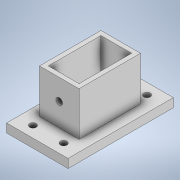
# Autodesk Inventor part: Lens Holder
Saved by Autodesk Inventor 2022 (Build 260153000, 153)
## iProperties
Created: 2023-09-18
Part Number: Lens Holder
Material: Generic
Document SubType Name: Modeling
Designer: fouad
Density: 1 g/cm^3
Appearance: Default
Author: fouad
Autodesk Inventor part; units mm, degrees
ref_plane "YZ Plane" through (0, 0, 0) normal (1, 0, 0) x (0, 1, 0)
ref_plane "XZ Plane" through (0, 0, 0) normal (0, 1, 0) x (-1, 0, 0)
ref_plane "XY Plane" through (0, 0, 0) normal (0, 0, 1) x (1, 0, 0)
sketch "Sketch1" plane through (0, 0, 0) normal (0, 1, 0) x (-1, 0, 0)
  line L0 (7.074, 9.2769) -> (0.074, 9.2769)
  line L1 (0.074, 9.2769) -> (0.074, -2.7231)
  line L2 (0.074, -2.7231) -> (7.074, -2.7231)
  line L3 (7.074, -2.7231) -> (7.074, 9.2769)
  line L4 (5.324, 6.2769) -> (1.824, 6.2769)
  line L5 (1.824, 6.2769) -> (1.824, 0.2769)
  line L6 (1.824, 0.2769) -> (5.324, 0.2769)
  line L7 (5.324, 0.2769) -> (5.324, 6.2769)
  point P0 (0, 0)
  dimension "d0" = 7
  dimension "d1" = 12
  dimension "d28" = 1.75
  dimension "d29" = 1.75
  dimension "d30" = 3
  dimension "d31" = 3
  constraints: 16 end point, 4 parallel, 2 horizontal, 2 perpendicular
  measures "d0" distance of L2.end L1.end
  measures "d1" distance of L1.end L0.end
  measures "d28" distance between parallel lines of L7 L3
  measures "d29" distance between parallel lines of L1 L5
  measures "d30" distance between parallel lines of L6 L2
  measures "d31" distance between parallel lines of L0 L4
extrude "Extrusion1" add sketch "Sketch1" along normal blind 1
sketch "Sketch3" plane through (0, 1, 0) normal (0, 1, 0) x (1, 0, 0)
  circle A0 centre (-5.324, -8.0269) radius 0.375
  line L0 (-7.074, -9.2769) -> (-0.074, -9.2769) projected
  line L1 (-7.074, 2.7231) -> (-7.074, -9.2769) projected
  circle A1 centre (-1.824, -8.0269) radius 0.375
  circle A2 centre (-5.324, 1.4731) radius 0.375
  circle A3 centre (-1.824, 1.4731) radius 0.375
  point P0 (0, 0)
  dimension "d8" = 0.75
  dimension "d9" = 1.25
  dimension "d10" = 1.75
  dimension "d13" = 3.5
  dimension "d16" = 9.5
  constraints: 4 centre point, 1 horizontal, 1 vertical, 6 other
  measures "d8" diameter of A0
  measures "d9" distance from line of L0 A0.centre
  measures "d10" distance from line of L1 A0.centre
  measures "d13" distance of A0.centre A1.centre
  measures "d16" distance of A0.centre A2.centre
extrude "Extrusion3" cut sketch "Sketch3" against normal blind 5
sketch "Sketch7" plane through (0, 1, 0) normal (0, 1, 0) x (1, 0, 0)
  line L0 (-1.824, -6.2769) -> (-5.324, -6.2769) projected
  line L1 (-1.824, -0.2769) -> (-1.824, -6.2769) projected
  line L2 (-5.324, -6.2769) -> (-1.824, -6.2769)
  line L3 (-1.824, -6.2769) -> (-1.824, -0.2769)
  line L4 (-1.824, -0.2769) -> (-5.324, -0.2769)
  line L5 (-5.324, -0.2769) -> (-5.324, -6.2769)
  line L6 (-5.824, -6.7769) -> (-1.324, -6.7769)
  line L7 (-1.324, -6.7769) -> (-1.324, 0.2231)
  line L8 (-1.324, 0.2231) -> (-5.824, 0.2231)
  line L9 (-5.824, 0.2231) -> (-5.824, -6.7769)
  point P0 (0, 0)
  dimension "d32" = 0.5
  constraints: 16 end point, 4 parallel, 2 perpendicular, 1 horizontal, 3 other
  measures "d32" distance between parallel lines of L5 L9
extrude "Extrusion5" add sketch "Sketch7" along normal blind 5
sketch "Sketch8" plane through (-5.824, 1, 6.7769) normal (0, 0, 1) x (1, 0, 0)
  circle A0 centre (2.25, 2.625) radius 0.375
  line L0 (0, 5) -> (4.5, 5) projected
  line L1 (0, 0) -> (0, 5) projected
  point P0 (5.824, -1)
  dimension "d35" = 0.75
  dimension "d36" = 2
  dimension "d37" = 2.25
  constraints: 1 centre point
  measures "d35" diameter of A0
  measures "d36" distance edge to line of A0 L0
  measures "d37" distance from line of L1 A0.centre
extrude "Extrusion6" cut sketch "Sketch8" against normal through all
body "Solid1"
